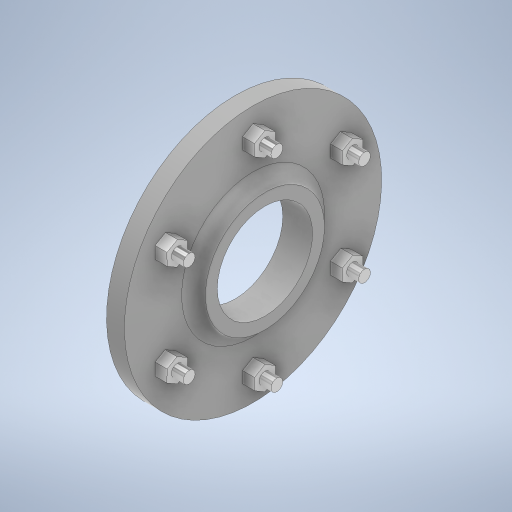
# Autodesk Inventor part: DN80-1m
Saved by Autodesk Inventor 2023 (Build 270158000, 158)
## iProperties
Created: 2024-11-14
Part Number: DN80-1m
Material: Generisch
Document SubType Name: Modeling
Designer: aurich
Density: 1 g/cm^3
Appearance: Vorgabe
Author: aurich
Autodesk Inventor part; units mm, degrees
ref_plane "YZ Plane" through (0, 0, 0) normal (1, 0, 0) x (0, 1, 0)
ref_plane "XZ Plane" through (0, 0, 0) normal (0, 1, 0) x (-1, 0, 0)
ref_plane "XY Plane" through (0, 0, 0) normal (0, 0, 1) x (1, 0, 0)
sketch "Skizze1" plane through (0, 0, 0) normal (1, 0, 0) x (0, 1, 0)
  circle A0 centre (0, 0) radius 40
  circle A1 centre (0, 0) radius 108
  dimension "d0" = 216
  dimension "d1" = 80
  constraints: 2 centre point, 2 coincident
  measures "d0" diameter of A1
  measures "d1" diameter of A0
extrude "Extrusion1" add sketch "Skizze1" along normal blind 15
sketch "Skizze2" plane through (15, 0, 0) normal (1, 0, 0) x (0, 0, -1)
  circle A0 centre (0, 0) radius 40
  circle A1 centre (0, 0) radius 50
  dimension "d4" = 100
  constraints: 2 centre point, 2 coincident
  measures "d4" diameter of A1
extrude "Extrusion2" add sketch "Skizze2" along normal blind 10
fillet "Rundung1" radius 10 1 edges at (15, 0, 50)
sketch "Skizze3" plane through (15, 0, 0) normal (1, 0, 0) x (0, 0, -1)
  circle A0 centre (0, -85) radius 10 construction
  line L0 (0, -95) -> (-8.7647, -89.8146)
  line L1 (-8.7647, -80.1854) -> (0, -75)
  line L2 (0, -75) -> (8.7647, -80.1854)
  line L3 (8.7647, -80.1854) -> (8.7647, -89.8146)
  line L4 (0, -95) -> (8.7647, -89.8146)
  line L5 (-8.7647, -80.1854) -> (-8.7647, -89.8146)
  point P0 (0, 0)
  dimension "d8" = 20
  dimension "d9" = 85
  constraints: 12 end point, 6 point on circle, 2 horizontal alignment, 2 parallel, 2 vertical alignment, 1 centre point, 1 vertical
  measures "d8" diameter of A0
  measures "d9" distance of point (0, 0) A0.centre
extrude "Extrusion3" add sketch "Skizze3" along normal blind 10
sketch "Skizze4" plane through (25, 0, 0) normal (1, 0, 0) x (0, 0, -1)
  circle A0 centre (0, -85) radius 5
  point P0 (0, 0)
  dimension "d12" = 10
  constraints: 1 centre point
  measures "d12" diameter of A0
extrude "Extrusion4" add sketch "Skizze4" along normal blind 10
pattern_circular "Runde Anordnung1" count 6 over 360 about axis through (-10, 0, 0) along (1, 0, 0) of "Extrusion3", "Extrusion4"
